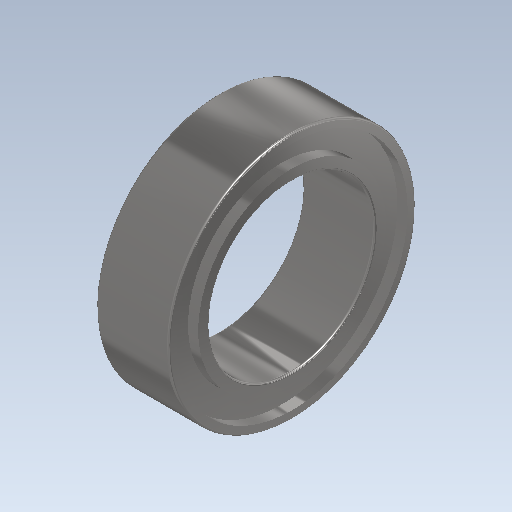
# Autodesk Inventor part: SB678ZZ
Saved by Autodesk Inventor 2021 (Build 250183000, 183)
## iProperties
Category: PARTsolutions
Company: MISUMI
Part Number: SB678ZZ
Material: ステンレス鋼
Catalog Web Link: www.cadenas.de
Description: B6 _ _ ZZ, B6 _ _ AZZ, SB6 _ _ ZZ, SB6 _ _ AZZ, BR _ _ ZZ, SBR _ _ ZZ-Small Ball Bearings - Double Shield Type
Vendor: MISUMI
Document SubType Name: Modeling
Designer: partserver
Manufacturer: MISUMI
Mass: 1.49196 g
Surface Area: 4.03318 cm^2
Volume: 0.186495 cm^3
Density: 8 g/cm^3
Appearance: 半つや出し
PSOL_IDENT_0: {$CADENAS_DATA\23d-libs\misumi\metric\12_bearing_holders\sb685zz.prj},221 {VTYP=3D},{NB=SB678ZZ},{LI
PSOL_IDENT_1: NA=SB678ZZ},{NN=B6 _ _ ZZ, B6 _ _ AZZ, SB6 _ _ ZZ, SB6 _ _ AZZ, BR _ _ ZZ, SBR _ _ ZZ},{DATE=09.09.2
PSOL_IDENT_2: 019 15:26:56},{GEOMDATE=23.07.2013 00:00:00},{VERSION=},{LINEID=150},{WBVAR=MAT},{WBNUMERIC=}  {NB=S
PSOL_IDENT_3: B678ZZ},{LINA=SB678ZZ},{KT=DUMMY},{PN=SB678ZZ},{MAT=S},{BN=678ZZ},{DD=8.0},{A=2.5100},{BB=0.400},{C=
PSOL_IDENT_4: 0.550},{D=12},{B=3.5},{RR=0.10},{CR=434},{COR=219},{CRS=543},{CRSS=434},{CORS=274},{CORSS=219},{DS=9
PSOL_IDENT_5: .05},{DDHH=11.33},{R=0.10},{MASS=0.99},{X=0},{BN2=B678ZZ}
NB: SB678ZZ
NN: B6 _ _ ZZ, B6 _ _ AZZ, SB6 _ _ ZZ, SB6 _ _ AZZ, BR _ _ ZZ, SBR _ _ ZZ
NT: Small Ball Bearings - Double Shield Type
NBSYN: $PN.
LINA: SB678ZZ
CATALOG: Misumi
PN: SB678ZZ
MAT: 440C Stainless Steel
BN: 678ZZ
DD: 8
D: 12
B: 3.5
RR: 0.1
CR: 434
COR: 219
DS: 9.05
DDHH: 11.33
R: 0.1
MASS: 0.99
X: 0
SUPPLIER: MISUMI
ARTICLENO: SB678ZZ
BOMINFO: SB678ZZ
CREATOR: CADENAS GmbH
d1: 0.000 mm
Title: SB678ZZ
Author: Cadenas PARTsolutions
Comments: Small Ball Bearings - Double Shield Type
Autodesk Inventor part; units mm, degrees
sketch "Sketch_1" plane through (0, 0, 0) normal (0, 0, 1) x (1, 0, 0)
  line L0 (3.4, 0) -> (0.1, 0)
  arc A0 (0, 4.1) -> (0.1, 4) centre (0.1, 4.1) ccw
  line L1 (0.1, 4) -> (3.4, 4)
  arc A1 (3.4, 4) -> (3.5, 4.1) centre (3.4, 4.1) ccw
  line L2 (3.5, 4.1) -> (3.5, 4.55)
  line L3 (3.5, 4.55) -> (3.005, 4.55)
  line L4 (3.005, 4.55) -> (3.005, 5.6)
  line L5 (3.005, 5.6) -> (3.5, 5.6)
  line L6 (3.5, 5.6) -> (3.5, 5.9)
  arc A2 (3.5, 5.9) -> (3.4, 6) centre (3.4, 5.9) ccw
  line L7 (3.4, 6) -> (0.1, 6)
  arc A3 (0.1, 6) -> (0, 5.9) centre (0.1, 5.9) ccw
  line L8 (0, 5.9) -> (0, 5.6)
  line L9 (0, 5.6) -> (0.495, 5.6)
  line L10 (0.495, 5.6) -> (0.495, 4.55)
  line L11 (0.495, 4.55) -> (0, 4.55)
  line L12 (0, 4.55) -> (0, 4.1)
  constraints: 26 end point, 8 point on circle, 4 centre point
revolve "Revolution1" add sketch "Sketch_1" angle 360 about axis through (3.4, 0, 0) along (1, 0, 0)
ref_plane "to_housing_XY" through (0, 0, 0) normal (1, 0, 0) x (0, 0, -1)
ref_plane "to_housing_YZ" through (0, 0, 0) normal (0, 0, -1) x (0, 1, 0)
ref_plane "to_housing_ZX" through (0, 0, 0) normal (0, 1, 0) x (1, 0, 0)
ref_plane "to_housing_center_XY" through (1.75, 0, 0) normal (1, 0, 0) x (0, 0, -1)
ref_plane "to_housing_center_YZ" through (1.75, 0, 0) normal (0, 0, -1) x (0, 1, 0)
ref_plane "to_housing_center_ZX" through (1.75, 0, 0) normal (0, 1, 0) x (1, 0, 0)
body "Solid1"
